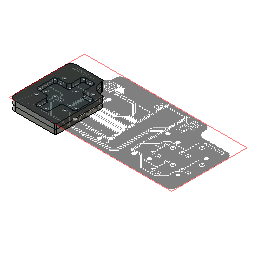
sprig_cover (Autodesk Fusion 360 design; units mm, degrees)
Autodesk Fusion 360 part; units mm, degrees
sketch "Sketch2" plane through (0, 0, 0) normal (0, 0, 1) x (1, 0, 0)
  line L0 (70.104, -32.512) -> (-70.104, -32.512)
  line L1 (-70.104, -32.512) -> (-70.104, 32.512)
  line L2 (-70.104, 32.512) -> (70.104, 32.512)
  line L3 (70.104, 32.512) -> (70.104, -32.512)
  line L4 (70.104, -32.512) -> (-70.104, 32.512) construction
  line L5 (-70.104, -32.512) -> (70.104, 32.512) construction
  dimension "d1" = 140.208
  dimension "d2" = 65.024
  constraint horizontal L0
  constraint perpendicular L0 L1
  constraint parallel L0 L2
  constraint parallel L1 L3
  constraint coincident L4 origin
  constraint coincident L5 origin
  measures "d1" distance of L1.end L2.end
  measures "d2" distance of L0.end L1.end
sketch "Sketch3" plane through (0, 0, 0) normal (0, 0, 1) x (1, 0, 0)
  line L0 (-70.104, 15.8) -> (-70.104, -27.3)
  arc A0 (-70.104, -27.3) -> (-64.904, -32.5) centre (-64.904, -27.3) ccw
  line L1 (-64.904, -32.5) -> (-30, -32.5)
  arc A1 (-64.904, 21) -> (-70.104, 15.8) centre (-64.904, 15.8) ccw
  line L2 (-64.904, 21) -> (-42, 21)
  line L3 (-30, 9) -> (-30, -32.5)
  circle A2 centre (-30.5373, 18.3875) radius 8
  line L4 (-30.5373, 22.2562) -> (-30.5373, 14.5188)
  line L5 (-42, 21) -> (-42, 19)
  arc A3 (-42, 19) -> (-32, 9) centre (-32, 19) ccw
  line L6 (-32, 9) -> (-30, 9)
  dimension "d3" = 70.104
  dimension "d4" = 32.5
  dimension "d5" = 5.2
  dimension "d6" = 21
  dimension "d7" = 5.2
  dimension "d8" = 16
  dimension "d9" = 42
  dimension "d10" = 9
  dimension "d11" = 10
  dimension "d12" = 30
  constraint vertical L0
  constraint tangent L0 A0
  constraint horizontal L1
  constraint tangent A0 L1
  constraint tangent L0 A1
  constraint horizontal L2
  constraint tangent A1 L2
  constraint perpendicular L2 L3
  constraint coincident L1.end L3.end
  constraint vertical L4
  constraint midpoint A2.centre L4
  constraint perpendicular L2 L5
  constraint tangent L5 A3
  constraint perpendicular L5 L6
  constraint tangent A3 L6
  measures "d3" distance of origin L0
  measures "d4" distance of origin L1
  measures "d5" radius of A0
  measures "d6" distance of origin L2
  measures "d7" radius of A1
  measures "d8" diameter of A2
  measures "d9" distance of origin L5
  measures "d10" distance of origin L6
  measures "d11" radius of A3
  measures "d12" distance of origin L3
extrude "Extrude1" add sketch "Sketch3" against normal blind 4 contours L0 A0 L1 A1 L2 L3 L5 A3 L6 makes body 1
fillet "Fillet3" radius 1 3 edges at (-30, -32.5, -2) (-30, 9, -2) (-42, 21, -2) on bodies 1
pattern_linear "R-Pattern1" count 2 spacing 4 along (0, 0, -1) of bodies 1 makes body 2
sketch "Sketch4" plane through (0, 0, 0) normal (0, 0, 1) x (-1, 0, 0)
  arc A0 (64.904, -21) -> (70.104, -15.8) centre (64.904, -15.8) ccw
  line L0 (70.104, -15.8) -> (70.104, 27.3)
  arc A1 (70.104, 27.3) -> (64.904, 32.5) centre (64.904, 27.3) ccw
  line L1 (64.904, 32.5) -> (31, 32.5)
  line L2 (30, 31.5) -> (30, -8)
  line L3 (31, -9) -> (32, -9)
  arc A2 (42, -19) -> (32, -9) centre (32, -19) ccw
  line L4 (42, -19) -> (42, -20)
  line L5 (43, -21) -> (64.904, -21)
  line L6 (65.35, -2.7) -> (48.35, -2.7)
  line L7 (48.35, -2.7) -> (48.35, 14.3)
  line L8 (48.35, 14.3) -> (65.35, 14.3)
  line L9 (65.35, 14.3) -> (65.35, -2.7)
  arc A3 (42, -20) -> (43, -21) centre (43, -20) ccw
  arc A4 (31, 32.5) -> (30, 31.5) centre (31, 31.5) ccw
  arc A5 (30, -8) -> (31, -9) centre (31, -8) ccw
  point P0 (48.35, 5.8)
  dimension "d21" = 5.8
  dimension "d22" = 17
  dimension "d23" = 48.35
  dimension "d24" = 17
  constraint horizontal L6
  constraint vertical L7
  constraint horizontal L8
  constraint vertical L9
  constraint midpoint L7 P0
  measures "d21" vertical distance of origin P0
  measures "d22" distance of L7.end L8.end
  measures "d23" horizontal distance of origin P0
  measures "d24" distance of L6.start L8.end
extrude "Extrude2" cut sketch "Sketch4" against normal blind 4 contours L6 L7 L8 L9 bodies 1
fillet "Fillet1" radius 2 2 edges at (-65.35, 2.7, -2) (-65.35, -14.3, -2) on bodies 1
mirror "Mirror1" about plane through (-48.35, 2.7, 0) normal (-1, 0, 0) of "Extrude2", "Fillet1"
sketch "Sketch5" plane through (0, 0, 0) normal (0, 0, 1) x (-1, 0, 0)
  line L0 (33.35, 14.3) -> (63.35, 14.3)
  arc A0 (65.35, 12.3) -> (63.35, 14.3) centre (63.35, 12.3) ccw
  line L1 (65.35, 12.3) -> (65.35, -0.7)
  arc A1 (63.35, -2.7) -> (65.35, -0.7) centre (63.35, -0.7) ccw
  line L2 (63.35, -2.7) -> (33.35, -2.7)
  arc A2 (31.35, -0.7) -> (33.35, -2.7) centre (33.35, -0.7) ccw
  line L3 (31.35, -0.7) -> (31.35, 12.3)
  arc A3 (33.35, 14.3) -> (31.35, 12.3) centre (33.35, 12.3) ccw
  arc A4 (42, -20) -> (43, -21) centre (43, -20) ccw
  line L4 (43, -21) -> (64.904, -21)
  arc A5 (64.904, -21) -> (70.104, -15.8) centre (64.904, -15.8) ccw
  line L5 (70.104, -15.8) -> (70.104, 27.3)
  arc A6 (70.104, 27.3) -> (64.904, 32.5) centre (64.904, 27.3) ccw
  line L6 (64.904, 32.5) -> (31, 32.5)
  arc A7 (31, 32.5) -> (30, 31.5) centre (31, 31.5) ccw
  line L7 (30, 31.5) -> (30, -8)
  arc A8 (30, -8) -> (31, -9) centre (31, -8) ccw
  line L8 (31, -9) -> (32, -9)
  arc A9 (42, -19) -> (32, -9) centre (32, -19) ccw
  line L9 (42, -19) -> (42, -20)
  line L10 (53.85, -2.7) -> (53.85, -15.2)
  line L11 (53.85, -15.2) -> (42.85, -15.2)
  line L12 (42.85, -15.2) -> (42.85, -2.7)
  point P0 (48.35, -2.7)
  point P1 (48.35, -15.2)
  dimension "d37" = 12.5
  dimension "d38" = 11
  constraint coincident L2 L10.start
  constraint perpendicular L2 L10
  constraint perpendicular L10 L11
  constraint coincident L2 L12.end
  constraint perpendicular L2 L12
  constraint midpoint L2 P0
  constraint midpoint L11 P1
  constraint vertical P0 P1
  measures "d37" distance of L11.end L12.end
  measures "d38" distance of L10.end L11.end
extrude "Extrude3" cut sketch "Sketch5" against normal blind 4 contours L2 L10 L11 L12 bodies 1
fillet "Fillet4" radius 2 2 edges at (-53.85, 15.2, -2) (-42.85, 15.2, -2) on bodies 1
ref_plane "WorkPlane1" through (-58.1, -5.8, -2) normal (0, -1, 0) x (-1, 0, 0)
mirror "Mirror2" about plane through (-58.1, -5.8, -2) normal (0, -1, 0) of "Extrude3", "Fillet4"
sketch "Sketch6" plane through (0, 0, 0) normal (0, 0, 1) x (-1, 0, 0)
  line L0 (53.85, 24.8) -> (53.85, 14.3)
  line L1 (53.85, 14.3) -> (63.35, 14.3)
  arc A0 (65.35, 12.3) -> (63.35, 14.3) centre (63.35, 12.3) ccw
  line L2 (65.35, 12.3) -> (65.35, -0.7)
  arc A1 (63.35, -2.7) -> (65.35, -0.7) centre (63.35, -0.7) ccw
  line L3 (63.35, -2.7) -> (53.85, -2.7)
  line L4 (53.85, -2.7) -> (53.85, -13.2)
  arc A2 (51.85, -15.2) -> (53.85, -13.2) centre (51.85, -13.2) ccw
  line L5 (51.85, -15.2) -> (44.85, -15.2)
  arc A3 (42.85, -13.2) -> (44.85, -15.2) centre (44.85, -13.2) ccw
  line L6 (42.85, -13.2) -> (42.85, -2.7)
  line L7 (42.85, -2.7) -> (33.35, -2.7)
  arc A4 (31.35, -0.7) -> (33.35, -2.7) centre (33.35, -0.7) ccw
  line L8 (31.35, -0.7) -> (31.35, 12.3)
  arc A5 (33.35, 14.3) -> (31.35, 12.3) centre (33.35, 12.3) ccw
  line L9 (33.35, 14.3) -> (42.85, 14.3)
  line L10 (42.85, 14.3) -> (42.85, 24.8)
  arc A6 (44.85, 26.8) -> (42.85, 24.8) centre (44.85, 24.8) ccw
  line L11 (44.85, 26.8) -> (51.85, 26.8)
  arc A7 (53.85, 24.8) -> (51.85, 26.8) centre (51.85, 24.8) ccw
  arc A8 (42, -20) -> (43, -21) centre (43, -20) ccw
  line L12 (43, -21) -> (64.904, -21)
  arc A9 (64.904, -21) -> (70.104, -15.8) centre (64.904, -15.8) ccw
  line L13 (70.104, -15.8) -> (70.104, 27.3)
  arc A10 (70.104, 27.3) -> (64.904, 32.5) centre (64.904, 27.3) ccw
  line L14 (64.904, 32.5) -> (31, 32.5)
  arc A11 (31, 32.5) -> (30, 31.5) centre (31, 31.5) ccw
  line L15 (30, 31.5) -> (30, -8)
  arc A12 (30, -8) -> (31, -9) centre (31, -8) ccw
  line L16 (31, -9) -> (32, -9)
  arc A13 (42, -19) -> (32, -9) centre (32, -19) ccw
  line L17 (42, -19) -> (42, -20)
  circle A14 centre (60.5272, -6.0993) radius 1.1
  circle A15 centre (36.0826, -6.0993) radius 1.1
  line L18 (60.5272, -6.0993) -> (36.0826, -6.0993) construction
  line L19 (36.0826, -6.0993) -> (36.0826, 18.3161) construction
  line L20 (36.0826, 18.3161) -> (60.5272, 18.3161) construction
  line L21 (60.5272, 18.3161) -> (60.5272, -6.0993) construction
  circle A16 centre (60.5272, 18.3161) radius 1.1
  circle A17 centre (36.0826, 18.3161) radius 1.1
  dimension "d45" = 2.2
  dimension "d46" = 2.2
  dimension "d47" = 2.2
  dimension "d48" = 2.2
  constraint horizontal L18
  constraint vertical L19
  constraint horizontal L20
  constraint vertical L21
  constraint coincident A14.centre L18.start
  constraint coincident A15.centre L18.end
  constraint coincident L20.end L21.start
  constraint coincident L19.end L20.start
  measures "d45" diameter of A14
  measures "d46" diameter of A15
  measures "d47" diameter of A16
  measures "d48" diameter of A17
extrude "Extrude4" cut sketch "Sketch6" against normal blind 18 contours A14 | A15 | A16 | A17 bodies 1 2
fillet "Fillet5" radius 2 4 edges at (-53.85, 2.7, -2) (-53.85, -14.3, -2) (-42.85, -14.3, -2) (-42.85, 2.7, -2) on bodies 1
sketch "Sketch10" plane through (0, 0, 0) normal (0, 0, 1) x (-1, 0, 0)
  arc A0 (42.85, -4.7) -> (40.85, -2.7) centre (40.85, -4.7) ccw
  line L0 (40.85, -2.7) -> (33.35, -2.7)
  arc A1 (31.35, -0.7) -> (33.35, -2.7) centre (33.35, -0.7) ccw
  line L1 (31.35, -0.7) -> (31.35, 12.3)
  arc A2 (33.35, 14.3) -> (31.35, 12.3) centre (33.35, 12.3) ccw
  line L2 (33.35, 14.3) -> (40.85, 14.3)
  arc A3 (40.85, 14.3) -> (42.85, 16.3) centre (40.85, 16.3) ccw
  line L3 (42.85, 16.3) -> (42.85, 24.8)
  arc A4 (44.85, 26.8) -> (42.85, 24.8) centre (44.85, 24.8) ccw
  line L4 (44.85, 26.8) -> (51.85, 26.8)
  arc A5 (53.85, 24.8) -> (51.85, 26.8) centre (51.85, 24.8) ccw
  line L5 (53.85, 24.8) -> (53.85, 16.3)
  arc A6 (53.85, 16.3) -> (55.85, 14.3) centre (55.85, 16.3) ccw
  line L6 (55.85, 14.3) -> (63.35, 14.3)
  arc A7 (65.35, 12.3) -> (63.35, 14.3) centre (63.35, 12.3) ccw
  line L7 (65.35, 12.3) -> (65.35, -0.7)
  arc A8 (63.35, -2.7) -> (65.35, -0.7) centre (63.35, -0.7) ccw
  line L8 (63.35, -2.7) -> (55.85, -2.7)
  arc A9 (55.85, -2.7) -> (53.85, -4.7) centre (55.85, -4.7) ccw
  line L9 (53.85, -4.7) -> (53.85, -13.2)
  arc A10 (51.85, -15.2) -> (53.85, -13.2) centre (51.85, -13.2) ccw
  line L10 (51.85, -15.2) -> (44.85, -15.2)
  arc A11 (42.85, -13.2) -> (44.85, -15.2) centre (44.85, -13.2) ccw
  line L11 (42.85, -13.2) -> (42.85, -4.7)
  circle A12 centre (60.5272, 18.3161) radius 1.1
  circle A13 centre (36.0826, 18.3161) radius 1.1
  circle A14 centre (60.5272, -6.0993) radius 1.1
  circle A15 centre (36.0826, -6.0993) radius 1.1
  arc A16 (42, -20) -> (43, -21) centre (43, -20) ccw
  line L12 (43, -21) -> (64.904, -21)
  arc A17 (64.904, -21) -> (70.104, -15.8) centre (64.904, -15.8) ccw
  line L13 (70.104, -15.8) -> (70.104, 27.3)
  arc A18 (70.104, 27.3) -> (64.904, 32.5) centre (64.904, 27.3) ccw
  line L14 (64.904, 32.5) -> (31, 32.5)
  arc A19 (31, 32.5) -> (30, 31.5) centre (31, 31.5) ccw
  line L15 (30, 31.5) -> (30, -8)
  arc A20 (30, -8) -> (31, -9) centre (31, -8) ccw
  line L16 (31, -9) -> (32, -9)
  arc A21 (42, -19) -> (32, -9) centre (32, -19) ccw
  line L17 (42, -19) -> (42, -20)
sketch "Sketch11" plane through (0, 0, -4) normal (0, 0, 1) x (-1, 0, 0)
  circle A0 centre (60.5272, 18.3161) radius 1.1
  circle A1 centre (36.0826, 18.3161) radius 1.1
  circle A2 centre (60.5272, -6.0993) radius 1.1
  circle A3 centre (36.0826, -6.0993) radius 1.1
  arc A4 (42, -20) -> (43, -21) centre (43, -20) ccw
  line L0 (43, -21) -> (64.904, -21)
  arc A5 (64.904, -21) -> (70.104, -15.8) centre (64.904, -15.8) ccw
  line L1 (70.104, -15.8) -> (70.104, 27.3)
  arc A6 (70.104, 27.3) -> (64.904, 32.5) centre (64.904, 27.3) ccw
  line L2 (64.904, 32.5) -> (31, 32.5)
  arc A7 (31, 32.5) -> (30, 31.5) centre (31, 31.5) ccw
  line L3 (30, 31.5) -> (30, -8)
  arc A8 (30, -8) -> (31, -9) centre (31, -8) ccw
  line L4 (31, -9) -> (32, -9)
  arc A9 (42, -19) -> (32, -9) centre (32, -19) ccw
  line L5 (42, -19) -> (42, -20)
equation "d3 = ( 140.208 / 2 ) * 1 mm"
